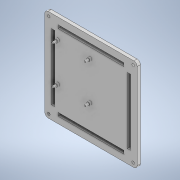
# Autodesk Inventor part: Led deksel niet hub
Saved by Autodesk Inventor 2021 (Build 250183000, 183)
## iProperties
Created: 2023-10-02
Part Number: Led deksel niet hub
Material: Generic
Document SubType Name: Modeling
Designer: Elias
Density: 1 g/cm^3
Appearance: Default
Author: Elias
Autodesk Inventor part; units mm, degrees
ref_plane "YZ Plane" through (0, 0, 0) normal (1, 0, 0) x (0, 1, 0)
ref_plane "XZ Plane" through (0, 0, 0) normal (0, 1, 0) x (-1, 0, 0)
ref_plane "XY Plane" through (0, 0, 0) normal (0, 0, 1) x (1, 0, 0)
sketch "Sketch1" plane through (0, 0, 0) normal (0, 0, 1) x (1, 0, 0)
  line L0 (0, 0) -> (140, 0)
  line L1 (140, 0) -> (140, 140)
  line L2 (140, 140) -> (0, 140)
  line L3 (0, 140) -> (0, 0)
  dimension "d0" = 140
  dimension "d1" = 140
  constraints: 8 end point, 2 parallel, 1 horizontal, 1 perpendicular
  measures "d0" distance of L1.end L2.end
  measures "d1" distance of L0.end L1.end
extrude "Extrusion1" add sketch "Sketch1" along normal blind 5
fillet "Fillet1" radius 5 4 edges at (140, 140, 2.5) (140, 0, 2.5) (0, 140, 2.5) (0, 0, 2.5)
sketch "Sketch2" plane through (0, 0, 5) normal (0, 0, 1) x (1, 0, 0)
  circle A0 centre (20, 110) radius 2.5
  line L0 (135, 140) -> (5, 140) projected
  line L1 (0, 135) -> (0, 5) projected
  circle A1 centre (69, 110) radius 2.5
  circle A2 centre (20, 52) radius 2.5
  circle A3 centre (69, 52) radius 2.5
  point P0 (0, 0)
  dimension "d5" = 5
  dimension "d6" = 30
  dimension "d7" = 20
  dimension "d8" = 5
  dimension "d9" = 30
  dimension "d10" = 69
  dimension "d11" = 5
  dimension "d12" = 20
  dimension "d13" = 88
  dimension "d14" = 5
  dimension "d15" = 88
  dimension "d16" = 69
  constraints: 4 centre point
  measures "d5" diameter of A0
  measures "d6" distance from line of L0 A0.centre
  measures "d7" distance from line of A0.centre L1
  measures "d8" diameter of A1
  measures "d9" distance from line of L0 A1.centre
  measures "d10" distance from line of L1 A1.centre
  measures "d11" diameter of A2
  measures "d12" distance from line of L1 A2.centre
  measures "d13" distance from line of L0 A2.centre
  measures "d14" diameter of A3
  measures "d15" distance from line of L0 A3.centre
  measures "d16" distance from line of L1 A3.centre
extrude "Extrusion2" add sketch "Sketch2" along normal blind 3
sketch "Sketch3" plane through (20, 110, 8) normal (0, 0, 1) x (1, 0, 0)
  circle A0 centre (0, 0) radius 1.35
  circle A1 centre (49, 0) radius 2.5 projected
  circle A2 centre (49, 0) radius 1.35
  circle A3 centre (0, -58) radius 2.5 projected
  circle A4 centre (0, -58) radius 1.35
  circle A5 centre (49, -58) radius 2.5 projected
  circle A6 centre (49, -58) radius 1.35
  point P0 (-20, -110)
  dimension "d19" = 2.7
  dimension "d20" = 2.7
  constraints: 4 centre point, 3 coincident
  measures "d19" diameter of A0
  measures "d20" diameter of A2
extrude "Extrusion3" add sketch "Sketch3" along normal blind 5 contours A0 | A2 | A4 | A6
sketch "Sketch4" plane through (0, 0, 5) normal (0, 0, 1) x (1, 0, 0)
  line L0 (135, 140) -> (5, 140) projected
  line L1 (0, 135) -> (0, 5) projected
  line L2 (140, 5) -> (140, 135) projected
  line L3 (5, 0) -> (135, 0) projected
  point P0 (0, 0)
  point P1 (6, 134)
  point P2 (134, 134)
  point P3 (6, 6)
  point P4 (134, 6)
  dimension "d30" = 6
  dimension "d31" = 6
  dimension "d32" = 6
  dimension "d33" = 6
  dimension "d34" = 6
  dimension "d35" = 6
  dimension "d36" = 6
  dimension "d37" = 6
  measures "d30" distance from line of L0 point (6, 134)
  measures "d31" distance from line of L1 point (6, 134)
  measures "d32" distance from line of L2 point (134, 134)
  measures "d33" distance from line of L0 point (134, 134)
  measures "d34" distance from line of L3 point (134, 6)
  measures "d35" distance from line of point (134, 6) L2
  measures "d36" distance from line of L1 point (6, 6)
  measures "d37" distance from line of L3 point (6, 6)
hole "Hole2" at (134, 134, 5) at (6, 6, 5) at (134, 6, 5) at (6, 134, 5) direction (0, 0, -1) diameter 4 depth 15
sketch "Sketch5" plane through (0, 0, 5) normal (0, 0, 1) x (1, 0, 0)
  line L0 (20, 130) -> (120, 130)
  line L1 (120, 130) -> (120, 125)
  line L2 (120, 125) -> (20, 125)
  line L3 (20, 125) -> (20, 130)
  line L4 (135, 140) -> (5, 140) projected
  line L5 (140, 5) -> (140, 135) projected
  line L6 (20, 15) -> (120, 15)
  line L7 (120, 15) -> (120, 10)
  line L8 (120, 10) -> (20, 10)
  line L9 (20, 10) -> (20, 15)
  line L10 (5, 0) -> (135, 0) projected
  line L11 (10, 120) -> (15, 120)
  line L12 (15, 120) -> (15, 20)
  line L13 (15, 20) -> (10, 20)
  line L14 (10, 20) -> (10, 120)
  line L15 (0, 135) -> (0, 5) projected
  line L16 (125, 120) -> (130, 120)
  line L17 (130, 120) -> (130, 20)
  line L18 (130, 20) -> (125, 20)
  line L19 (125, 20) -> (125, 120)
  point P0 (0, 0)
  dimension "d45" = 10
  dimension "d46" = 5
  dimension "d47" = 20
  dimension "d48" = 100
  dimension "d49" = 100
  dimension "d50" = 5
  dimension "d51" = 20
  dimension "d52" = 10
  dimension "d53" = 5
  dimension "d54" = 100
  dimension "d55" = 20
  dimension "d56" = 10
  dimension "d57" = 5
  dimension "d58" = 100
  dimension "d59" = 10
  dimension "d60" = 20
  constraints: 32 end point, 8 parallel, 4 horizontal, 4 perpendicular
  measures "d45" distance between parallel lines of L4 L0
  measures "d46" distance of L0.end L1.end
  measures "d47" distance between parallel lines of L5 L1
  measures "d48" distance of L0.start L0.end
  measures "d49" distance of L6.start L6.end
  measures "d50" distance of L6.end L7.end
  measures "d51" distance from line of L5 L6.end
  measures "d52" distance between parallel lines of L10 L8
  measures "d53" distance of L11.start L11.end
  measures "d54" distance of L11.end L12.end
  measures "d55" distance between parallel lines of L10 L13
  measures "d56" distance between parallel lines of L15 L14
  measures "d57" distance of L16.start L16.end
  measures "d58" distance of L16.end L17.end
  measures "d59" distance between parallel lines of L5 L17
  measures "d60" distance between parallel lines of L10 L18
extrude "Extrusion4" cut sketch "Sketch5" against normal blind 10
body "Solid1"
